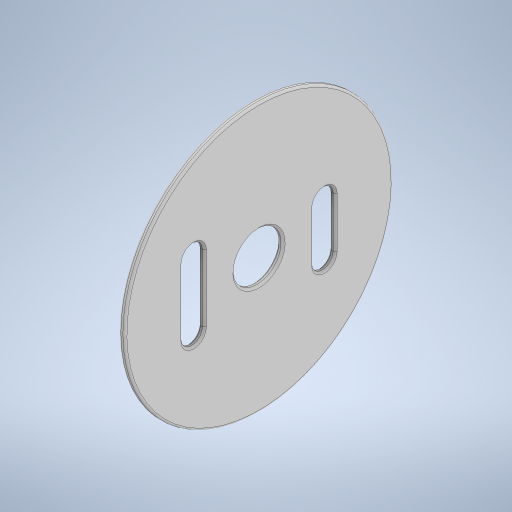
# Autodesk Inventor part: CameraModuleSymbolDisc
Saved by Autodesk Inventor 2023 (Build 270158000, 158)
## iProperties
Created: 2026-02-09
Part Number: CameraModuleSymbolDisc
Material: Generic
Document SubType Name: Modeling
Designer: DanAr
Density: 1 g/cm^3
Appearance: Default
Author: DanAr
Autodesk Inventor part; units mm, degrees
ref_plane "YZ Plane" through (0, 0, 0) normal (1, 0, 0) x (0, 1, 0)
ref_plane "XZ Plane" through (0, 0, 0) normal (0, 1, 0) x (-1, 0, 0)
ref_plane "XY Plane" through (0, 0, 0) normal (0, 0, 1) x (1, 0, 0)
sketch "Sketch1" plane through (0, 0, 0) normal (1, 0, 0) x (0, 1, 0)
  circle A0 centre (0, 0) radius 3.6
  line L0 (-5, -9.75) -> (5, -9.75)
  line L1 (5, -9.75) -> (5, 9.75)
  line L2 (5, 9.75) -> (-5, 9.75)
  line L3 (-5, 9.75) -> (-5, -9.75)
  line L4 (-5, -9.75) -> (5, 9.75) construction
  line L5 (5, -9.75) -> (-5, 9.75) construction
  line L6 (5, 9.75) -> (-5, 9.75) construction
  line L7 (5, 11.35) -> (-5, 11.35)
  line L8 (-5, 8.15) -> (5, 8.15)
  arc A1 (5, 8.15) -> (5, 11.35) centre (5, 9.75) ccw
  arc A2 (-5, 11.35) -> (-5, 8.15) centre (-5, 9.75) ccw
  line L9 (-5, -9.75) -> (2.5, -9.75) construction
  line L10 (-5, -11.35) -> (2.5, -11.35)
  line L11 (2.5, -8.15) -> (-5, -8.15)
  arc A3 (-5, -8.15) -> (-5, -11.35) centre (-5, -9.75) ccw
  arc A4 (2.5, -11.35) -> (2.5, -8.15) centre (2.5, -9.75) ccw
  circle A5 centre (0, 0) radius 20
  point P0 (0, 9.75)
  point P1 (-1.25, -9.75)
  dimension "d0" = 7.2
  dimension "d1" = 19.5
  dimension "d2" = 10
  dimension "d3" = 1.6
  dimension "d4" = 7.5
  dimension "d5" = 40
  dimension "d12" = 1.6
  constraints: 28 end point, 8 point on circle, 8 tangent, 6 centre point, 5 equal length, 4 midpoint, 2 coincident, 1 horizontal, 1 perpendicular, 1 point on line
  measures "d0" diameter of A0
  measures "d1" distance of L0.end L1.end
  measures "d2" distance of L1.end L2.end
  measures "d3" radius of A1
  measures "d4" distance of L10.start L10.end
  measures "d5" diameter of A5
  measures "d12" radius of A3
extrude "Extrusion1" add sketch "Sketch1" along normal blind 0.9 contours A4 L11 L3 L8 L1 L0 | A5
fillet "Fillet1" radius 0.3 2 edges at (0.9, -20, 0) (0, -20, 0)
chamfer "Chamfer1" distance 0.3 angle 45 18 edges at (0.9, 0, 8.15) (0.9, -6.6, 9.75) (0.9, 0, 11.35) (0.9, 6.6, 9.75) (0.9, -3.6, 0) (0, -3.6, 0) (0, -1.25, -11.35) (0, -6.6, -9.75) (0, -1.25, -8.15) (0, 4.1, -9.75) (0.9, -1.25, -11.35) (0.9, -6.6, -9.75) (0.9, -1.25, -8.15) (0.9, 4.1, -9.75) (0, 0, 8.15) (0, -6.6, 9.75) (0, 0, 11.35) (0, 6.6, 9.75)
body "Solid1"
